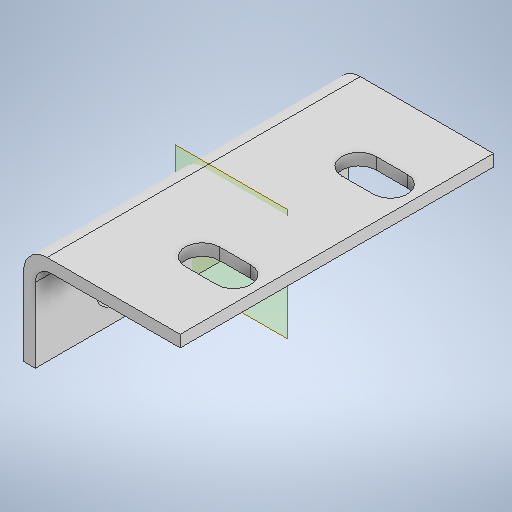
# Autodesk Inventor part: Winkelblech
Saved by Autodesk Inventor 2025.2 (Build 292293000, 293)
## iProperties
Created: 2025-06-22
Part Number: Winkelblech
Material: Generisch
Document SubType Name: Sheet Metal
Designer: Jakob
Density: 1 g/cm^3
Sheet Metal Rule: Standard_mm
Appearance: Vorgabe
Author: Jakob
Autodesk Inventor part; units mm, degrees
sketch "Skizze1" plane through (0, 0, 0) normal (0, 1, 0) x (-1, 0, 0)
  line L0 (0, 0) -> (-3, 0)
  line L1 (-3, 0) -> (-3, 23)
  line L2 (-3, 23) -> (-40, 23)
  line L3 (-40, 23) -> (-40, 26)
  line L4 (-40, 26) -> (0, 26)
  line L5 (0, 26) -> (0, 0)
  line L6 (0, -5.2) -> (0, 31.2) projected
  line L7 (8, 0) -> (-48, 0) projected
  point P0 (0, 0)
  dimension "d0" = 3
  dimension "d1" = 3
  dimension "d2" = 40
  dimension "d3" = 26
  constraints: 12 end point, 4 perpendicular, 2 collinear, 1 horizontal, 1 parallel
  measures "d0" distance between parallel lines of L2 L4
  measures "d1" distance between parallel lines of L5 L1
  measures "d2" distance between parallel lines of L3 L5
  measures "d3" distance between parallel lines of L0 L4
extrude "Extrusion1" add sketch "Skizze1" along normal blind 80
fillet "Rundung1" radius 6 1 edges at (0, 40, 26)
fillet "Rundung2" radius 4 1 edges at (3, 40, 23)
sketch "Skizze2" plane through (3, 0, 0) normal (1, 0, 0) x (0, 0, -1)
  arc A0 (-14.35, 24.35) -> (-14.35, 15.65) centre (-14.35, 20) ccw
  arc A1 (-8.35, 15.65) -> (-8.35, 24.35) centre (-8.35, 20) ccw
  line L0 (-14.35, 24.35) -> (-8.35, 24.35)
  line L1 (-8.35, 15.65) -> (-14.35, 15.65)
  line L2 (-31.2, 0) -> (5.2, 0) projected
  line L3 (0, 0) -> (0, 80) projected
  point P0 (-4, 20)
  dimension "d17" = 8.7
  dimension "d18" = 6
  dimension "d19" = 20
  dimension "d20" = 8.7
  dimension "d21" = 4
  constraints: 5 point on circle, 4 end point, 2 centre point, 2 tangent, 1 equal radius, 1 horizontal, 1 parallel
  measures "d17" diameter of A0
  measures "d18" distance of A1.centre A0.centre
  measures "d19" distance from line of L2 A1.centre
  measures "d20" distance between parallel lines of L0 L1
  measures "d21" distance from line of L3 point (-4, 20)
extrude "Extrusion2" cut sketch "Skizze2" against normal through all
ref_plane "Arbeitsebene1" through (0, 40, 0) normal (0, 1, 0) x (-1, 0, 0)
mirror "Spiegeln1" about plane through (0, 40, 0) normal (0, 1, 0) of "Extrusion2"
sketch "Skizze3" plane through (40, 0, 23) normal (0, 0, -1) x (-1, 0, 0)
  arc A0 (6.35, 24.35) -> (6.35, 15.65) centre (6.35, 20) ccw
  arc A1 (14.35, 15.65) -> (14.35, 24.35) centre (14.35, 20) ccw
  line L0 (6.35, 24.35) -> (14.35, 24.35)
  line L1 (14.35, 15.65) -> (6.35, 15.65)
  line L2 (48, 0) -> (-8, 0) projected
  line L3 (0, 0) -> (0, 80) projected
  point P0 (40, 0)
  point P1 (2, 20)
  dimension "d23" = 8.7
  dimension "d24" = 8
  dimension "d25" = 20
  dimension "d26" = 2
  constraints: 5 point on circle, 4 end point, 4 tangent, 2 centre point, 1 equal radius, 1 horizontal
  measures "d23" diameter of A0
  measures "d24" distance of A1.centre A0.centre
  measures "d25" distance from line of L2 A1.centre
  measures "d26" distance from line of L3 point (2, 20)
extrude "Extrusion3" cut sketch "Skizze3" against normal blind 10
mirror "Spiegeln2" about plane through (0, 40, 0) normal (0, 1, 0) of "Extrusion3"
ref_plane "Arbeitsebene2" through (3, 20, 8.35) normal (0, -1, 0) x (1, 0, 0)
ref_plane "Arbeitsebene3" through (0, 60, 8.35) normal (0, -1, 0) x (1, 0, 0)
ref_plane "Arbeitsebene4" through (3, 0, 11.35) normal (0, 0, -1) x (-1, 0, 0)
ref_plane "Arbeitsebene5" through (0, 20, 0) normal (0, -1, 0) x (1, 0, 0)
ref_plane "Arbeitsebene6" through (0, 60, 0) normal (0, 1, 0) x (1, 0, 0)
ref_plane "Arbeitsebene7" through (29.65, 0, 26) normal (1, 0, 0) x (0, 0, -1)
equation "\"Biegeradius\" = Stärke"
equation "\"BreiteBiegungsfreistellung\" = Stärke"
equation "\"TiefeBiegungsfreistellung\" = 0.5 * Stärke"
equation "\"GrößeEckenfreistellung\" = 4 * Stärke"
equation "\"MinimalRest\" = 2 * Stärke"
equation "\"Übergangsradius\" = Biegeradius"
equation "\"JacobiRadiusGröße\" = Biegeradius"
equation "\"Abstandsgröße\" = Stärke"
equation "\"Stärke\" = 0.5"
